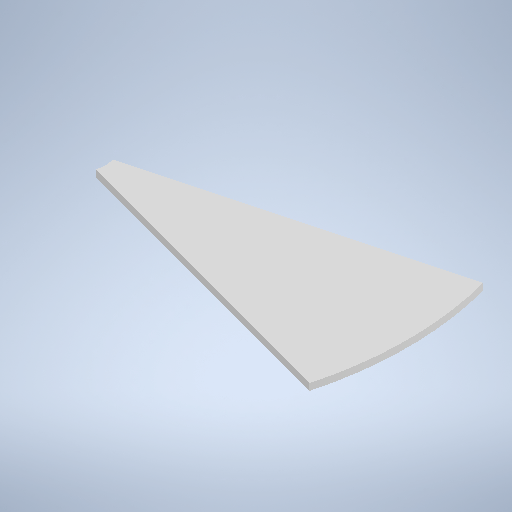
# Autodesk Inventor part: PTFE_Cut_Guide
Saved by Autodesk Inventor 2025.1 (Build 291241000, 241)
## iProperties
Created: 2026-04-28
Part Number: PTFE_Cut_Guide
Material: Generic
Document SubType Name: Modeling
Designer: ryand
Density: 1 g/cm^3
Appearance: Default
Author: ryand
Autodesk Inventor part; units mm, degrees
ref_plane "YZ Plane" through (0, 0, 0) normal (1, 0, 0) x (0, 1, 0)
ref_plane "XZ Plane" through (0, 0, 0) normal (0, 1, 0) x (-1, 0, 0)
ref_plane "XY Plane" through (0, 0, 0) normal (0, 0, 1) x (1, 0, 0)
sketch "Sketch3" plane through (0, 0, 0) normal (0, 1, 0) x (-1, 0, 0)
  arc A0 (0.1704, 1.2941) -> (0.1704, -1.2941) centre (5, 0) ccw
  arc A1 (-43.2963, 12.941) -> (-43.2963, -12.941) centre (5, 0) ccw
  line L0 (0.1704, -1.2941) -> (-43.2963, -12.941)
  line L1 (0.1704, 1.2941) -> (-43.2963, 12.941)
  point P0 (0, 0)
  point P1 (0, 0)
  dimension "d6" = 5
  dimension "d7" = 50
  dimension "d8" = 0
  dimension "d9" = 0
  constraints: 5 point on circle, 4 end point, 2 centre point
  measures "d6" radius of A0
  measures "d7" radius of A1
  measures "d8" distance of point (0, 0) point (0, 0)
  measures "d9" distance of point (0, 0) point (0, 0)
extrude "Extrusion2" add sketch "Sketch3" along normal blind 1
body "Solid2"
